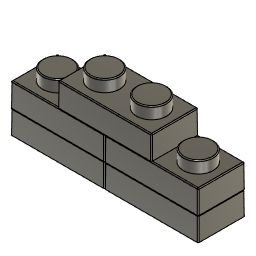
Building Blocks - PE (Autodesk Fusion 360 design; units mm, degrees)
Autodesk Fusion 360 part; units mm, degrees
sketch "Sketch1" plane through (0, 0, 0) normal (0, 0, 1) x (1, 0, 0)
  line L0 (12.5, -6.25) -> (-12.5, -6.25)
  line L1 (-12.5, -6.25) -> (-12.5, 6.25)
  line L2 (-12.5, 6.25) -> (12.5, 6.25)
  line L3 (12.5, 6.25) -> (12.5, -6.25)
  line L4 (12.5, -6.25) -> (-12.5, 6.25) construction
  line L5 (-12.5, -6.25) -> (12.5, 6.25) construction
  dimension "d1" = 25
  dimension "d2" = 12.5
  constraint perpendicular L0 L1
  constraint parallel L0 L2
  constraint parallel L1 L3
  constraint horizontal L0
  constraint coincident L4 origin
  constraint coincident L5 origin
  measures "d1" distance of L1.end L2.end
  measures "d2" distance of L0.end L1.end
extrude "Extrude1" add sketch "Sketch1" along normal blind 6.25 draft -0.5 makes body 1
sketch "Sketch2" plane through (0, 0, 6.25) normal (0, 0, 1) x (-1, 0, 0)
  line L0 (-12.4455, 6.1955) -> (-12.4455, -6.1955)
  line L1 (-12.4455, -6.1955) -> (12.4455, -6.1955)
  line L2 (12.4455, -6.1955) -> (12.4455, 6.1955)
  line L3 (12.4455, 6.1955) -> (-12.4455, 6.1955)
  line L4 (6.25, 0) -> (-6.25, 0) construction
  circle A0 centre (-6.25, 0) radius 4
  circle A1 centre (6.25, 0) radius 4
  dimension "d5" = 12.5
  dimension "d6" = 8
  constraint horizontal L4
  constraint midpoint origin L4
  constraint coincident L4.end A0.centre
  constraint coincident L4.start A1.centre
  constraint equal A0 A1
  measures "d5" distance of L4.start L4.end
  measures "d6" diameter of A0
extrude "Extrude2" add sketch "Sketch2" along normal blind 3.1 draft -0.5 contours A0 | A1 bodies 1
fillet "Fillet1" radius 0.25 10 edges at (12.4727, -6.2227, 3.125) (12.4727, 6.2227, 3.125) (12.4455, 0, 6.25) (0, 6.1955, 6.25) (0, -6.1955, 6.25) (-12.4727, 6.2227, 3.125) (-12.4727, -6.2227, 3.125) (-12.4455, 0, 6.25) (-2.5459, -1.4367, 9.35) (9.9541, -1.4367, 9.35) on bodies 1
shell "Shell1" thickness 0.5 removed faces 1 at (4.0833, -2.0833, 0) on bodies 1
sketch "Sketch3" plane through (0, 0, 0) normal (0, 0, -1) x (1, 0, 0)
  line L0 (-12, 5.75) -> (12, 5.75)
  line L1 (12, 5.75) -> (12, -5.75)
  line L2 (12, -5.75) -> (-12, -5.75)
  line L3 (-12, -5.75) -> (-12, 5.75)
  ellipse E0 centre (-12.25, -6) end of major axis (-12.4268, -6.1768) minor radius 0.25 (-12.5, -6) -> (-12.25, -6.25) ccw
  line L4 (-12.25, -6.25) -> (12.25, -6.25)
  ellipse E1 centre (12.25, -6) end of major axis (12.4268, -6.1768) minor radius 0.25 (12.25, -6.25) -> (12.5, -6) ccw
  line L5 (12.5, -6) -> (12.5, 6)
  ellipse E2 centre (12.25, 6) end of major axis (12.4268, 6.1768) minor radius 0.25 (12.5, 6) -> (12.25, 6.25) ccw
  line L6 (12.25, 6.25) -> (-12.25, 6.25)
  ellipse E3 centre (-12.25, 6) end of major axis (-12.4268, 6.1768) minor radius 0.25 (-12.25, 6.25) -> (-12.5, 6) ccw
  line L7 (-12.5, 6) -> (-12.5, -6)
  circle A0 centre (-6.25, 0) radius 4
  circle A1 centre (6.25, 0) radius 4
  line L8 (0, 5.75) -> (0, -5.75) construction
  line L9 (6, 5.75) -> (6.5, 5.75)
  line L10 (6.5, 5.75) -> (6.5, 3.9922)
  line L11 (6.5, 3.9922) -> (6, 3.9922)
  line L12 (6, 3.9922) -> (6, 5.75)
  line L13 (10.2422, 0.25) -> (12, 0.25)
  line L14 (12, 0.25) -> (12, -0.25)
  line L15 (12, -0.25) -> (10.2422, -0.25)
  line L16 (10.2422, -0.25) -> (10.2422, 0.25)
  line L17 (0, 0) -> (4.6754, 0) construction
  line L18 (6.25, 3.9922) -> (6.25, 0) construction
  line L19 (6.25, 0) -> (10.2422, 0) construction
  line L20 (6.5, -5.75) -> (6.5, -3.9922)
  line L21 (6, -3.9922) -> (6, -5.75)
  line L22 (6, -5.75) -> (6.5, -5.75)
  line L23 (6.5, -3.9922) -> (6, -3.9922)
  dimension "d11" = 0.5
  dimension "d12" = 0.5
  constraint midpoint L0 L8.start
  constraint midpoint L2 L8.end
  constraint horizontal L9
  constraint vertical L10
  constraint horizontal L11
  constraint vertical L12
  constraint coincident A1 L10.end
  constraint coincident L0 L9.start
  constraint horizontal L13
  constraint vertical L14
  constraint horizontal L15
  constraint vertical L16
  constraint coincident L1 L14.end
  constraint coincident A1 L13.start
  constraint coincident L17.start origin
  constraint perpendicular L8 L17
  constraint midpoint L11 L18.start
  constraint coincident A1.centre L18.end
  constraint midpoint L16 L19.end
  constraint horizontal L19
  constraint vertical L18
  constraint symmetric L9.start L19 L21.end
  constraint symmetric L9.end L19 L20.start
  constraint symmetric L10.end L19 L20.end
  constraint symmetric L11.end L19 L21.start
  measures "d11" distance of L9.start L9.end
  measures "d12" distance of L13.end L14.end
extrude "Extrude3" add sketch "Sketch3" against normal up to surface (5.75 mm away) draft 0.5 contours L0 A1 L9 L10 L12 | A1 L11 | L2 A1 L20 L21 L22 | A1 L23 | L1 A1 L13 L14 L15 | A1 L16 bodies 1
mirror "Mirror1" about plane through (0, 0, 0) normal (1, 0, 0) of "Extrude3"
copy_body "CopyPasteBodies1" bodies 1 makes body 2
move_body "Move1" bodies 2 to x (1, 0, 0) y (0, 1, 0) z (0, 0, 1) at (0, 0, 6.25)
copy_body "CopyPasteBodies2" bodies 2 makes body 3
move_body "Move2" bodies 3 to x (1, 0, 0) y (0, 1, 0) z (0, 0, 1) at (12.5, 0.0545, 6.2498)
copy_body "CopyPasteBodies3" bodies 1 2 makes body 4 makes body 5
move_body "Move3" bodies 4 5 to x (1, 0, 0) y (0, 1, 0) z (0, 0, 1) at (25, 0, 0)
equation "d7 = ( 12.4 / 4 ) * 1 mm"
equation "d12 = d11"
